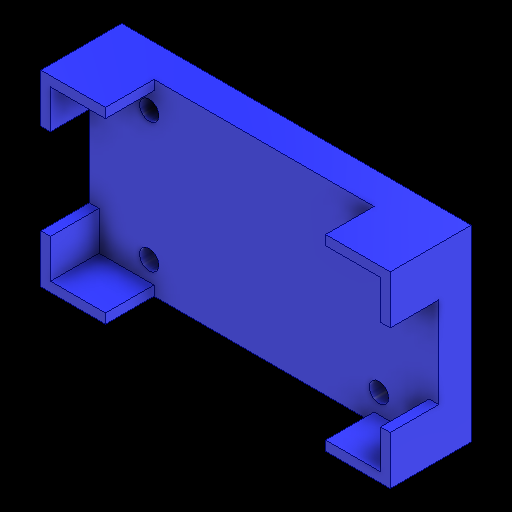
# Autodesk Inventor part: magnet_holder
Saved by Autodesk Inventor 2026.1 (Build 301233000, 233)
## iProperties
Created: 2025-09-30
Part Number: magnet_holder
Material: PC/ABS Plastic
Document SubType Name: Modeling
Designer: drago
Density: 1.1 g/cm^3
Appearance: Blue - Wall Paint - Glossy
Author: drago
Autodesk Inventor part; units mm, degrees
ref_plane "YZ Plane" through (0, 0, 0) normal (1, 0, 0) x (0, 1, 0)
ref_plane "XZ Plane" through (0, 0, 0) normal (0, 1, 0) x (-1, 0, 0)
ref_plane "XY Plane" through (0, 0, 0) normal (0, 0, 1) x (1, 0, 0)
sketch "Sketch1" plane through (0, 0, 0) normal (0, 0, 1) x (1, 0, 0)
  line L0 (54, -29) -> (-54, -29)
  line L1 (-54, -29) -> (-54, 29)
  line L2 (-54, 29) -> (54, 29)
  line L3 (54, 29) -> (54, -29)
  line L4 (51, -26) -> (-51, -26)
  line L5 (-51, -26) -> (-51, 26)
  line L6 (-51, 26) -> (51, 26)
  line L7 (51, 26) -> (51, -26)
  line L8 (54, 0) -> (-54, 0) construction
  line L9 (0, -29) -> (0, 29) construction
  line L10 (-34, 29) -> (-34, 26)
  line L11 (-54, 14) -> (-51, 14)
  line L12 (34, -26) -> (34, -29)
  line L13 (51, -14) -> (54, -14)
  line L14 (-34, -26) -> (-34, -29)
  line L15 (-54, -14) -> (-51, -14)
  line L16 (34, 29) -> (34, 26)
  line L17 (51, 14) -> (54, 14)
  point P0 (0, 0)
  point P1 (-35.5, 20)
  point P2 (35.5, 20)
  point P3 (35.5, -20)
  point P4 (-35.5, -20)
  dimension "d0" = 108
  dimension "d1" = 58
  dimension "d2" = 102
  dimension "d3" = 52
  dimension "d4" = 15
  dimension "d5" = 20
  dimension "d6" = 40
  dimension "d7" = 71
  constraints: 36 end point, 16 point on line, 11 perpendicular, 4 collinear, 4 midpoint, 4 parallel, 3 symmetric about line, 2 horizontal, 5 other
  measures "d0" distance of L1.end L2.end
  measures "d1" distance between parallel lines of L0 L2
  measures "d2" distance of L5.end L6.end
  measures "d3" distance of L4.end L5.end
  measures "d4" distance between parallel lines of L0 L13
  measures "d5" distance between parallel lines of L3 L12
  measures "d6" distance of point (35.5, 20) point (35.5, -20)
  measures "d7" distance of point (35.5, -20) point (-35.5, -20)
extrude "Extrusion1" add sketch "Sketch1" against normal blind 10
extrude "Extrusion2" add sketch "Sketch1" along normal blind 15 contours L0 L12 L4 L7 L13 L3 | L0 L1 L15 L5 L4 L14 | L17 L7 L6 L16 L2 L3 | L1 L2 L10 L6 L5 L11
hole "Hole1" at (-35.5, 20, 0) at (35.5, 20, 0) at (35.5, -20, 0) at (-35.5, -20, 0) direction (0, 0, -1) diameter 3.5 end through all counterbore diameter 6 counterbore depth 5
equation "\"d0\" = magnet_length + 2 * delta"
equation "\"d1\" = magnet_width + 2 * delta"
equation "\"d2\" = magnet_length"
equation "\"d3\" = magnet_width"
equation "\"magnet_width\" = 52"
equation "\"magnet_length\" = 102"
equation "\"delta\" = 3"
body "Solid1"
